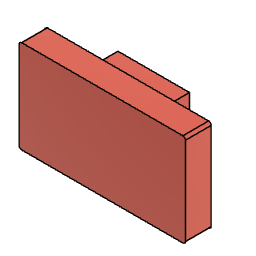
Switch Blocker v1 (Autodesk Fusion 360 design; units mm, degrees)
Autodesk Fusion 360 part; units mm, degrees
sketch "Sketch1" plane through (0, 0, 0) normal (0, 1, 0) x (1, 0, 0)
  line L0 (25.1, -18.075) -> (-6.2375, -18.075)
  line L1 (-6.7375, -17.575) -> (-6.7375, -0.525)
  line L2 (-6.2375, -0.025) -> (25.1, -0.025)
  line L3 (25.6, -17.575) -> (25.6, -0.525)
  line L4 (16.3813, -16) -> (16.3813, -2.1)
  line L5 (2.4813, -2.1) -> (16.3813, -2.1)
  line L6 (2.4813, -16) -> (2.4813, -2.1)
  line L7 (16.3813, -16) -> (2.4813, -16)
  arc A0 (-6.7375, -17.575) -> (-6.2375, -18.075) centre (-6.2375, -17.575) ccw
  arc A1 (-6.2375, -0.025) -> (-6.7375, -0.525) centre (-6.2375, -0.525) ccw
  arc A2 (25.1, -18.075) -> (25.6, -17.575) centre (25.1, -17.575) ccw
  arc A3 (25.6, -0.525) -> (25.1, -0.025) centre (25.1, -0.525) ccw
  line L8 (8.8409, -16) -> (8.8409, -18.075)
  line L9 (16.3813, -6.6239) -> (25.6, -6.6239)
  point P0 (25.6, -18.075)
  point P1 (-6.7375, -18.075)
  point P2 (25.6, -0.025)
  dimension "d39" = 0.5
  dimension "d40" = 0.5
  dimension "d41" = 0.5
  dimension "d42" = 0.5
  dimension "StemWidth" = 13.9
  dimension "StemHeight" = 13.9
  dimension "d62" = 2.075
  dimension "d63" = 9.2188
  constraint horizontal L0
  constraint vertical L1
  constraint horizontal L2
  constraint perpendicular L2 L3
  constraint coincident P1 L0
  constraint coincident P1 L1
  constraint tangent L0 A0
  constraint tangent L1 A0
  constraint tangent L1 A1
  constraint tangent L2 A1
  constraint coincident P0 L0
  constraint coincident P0 L3
  constraint tangent L0 A2
  constraint tangent L3 A2
  constraint coincident P2 L2
  constraint coincident P2 L3
  constraint tangent L2 A3
  constraint tangent L3 A3
  constraint parallel L3 L4
  constraint parallel L2 L5
  constraint parallel L1 L6
  constraint parallel L0 L7
  constraint coincident L7 L8.start
  constraint coincident L0 L8.end
  constraint perpendicular L0 L8
  constraint coincident L4 L9.start
  constraint coincident L3 L9.end
  constraint perpendicular L3 L9
  measures "d39" radius of A0
  measures "d40" radius of A1
  measures "d41" radius of A2
  measures "d42" radius of A3
  measures "StemWidth" distance of L4.start L4.end
  measures "StemHeight" distance of L4.start L6.start
  measures "d62" distance of L8.start L8.end
  measures "d63" distance of L9.start L9.end
extrude "Extrude1" add sketch "Sketch1" against normal blind 2
extrude "Extrude2" add sketch "Sketch1" along normal blind 5 contours L4 L5 L6 L7
extrude "Extrude3" add 1 faces at (4.2083, -2, 6.0417) along direction (0, -1, 0) blind 3
sketch "Sketch2" plane through (16.3813, 0, 0) normal (1, 0, 0) x (0, 1, 0)
  line L0 (0, 16) -> (0, 2.1)
  line L1 (0, 2.1) -> (5, 2.1)
  line L2 (5, 2.1) -> (5, 16)
  line L3 (5, 16) -> (0, 16)
  line L4 (0, 16) -> (0, 14)
  line L5 (0, 2.1) -> (0, 4.1)
  line L6 (0, 14) -> (1.5, 14)
  line L7 (0, 4.1) -> (1.5, 4.1)
  line L8 (1.5, 14) -> (3.5, 14)
  line L9 (3.5, 14) -> (3.5, 13)
  line L10 (3.5, 13) -> (1.5, 13)
  line L11 (1.5, 13) -> (1.5, 14)
  line L12 (1.5, 4.1) -> (3.5, 4.1)
  line L13 (3.5, 4.1) -> (3.5, 5.1)
  line L14 (3.5, 5.1) -> (1.5, 5.1)
  line L15 (1.5, 5.1) -> (1.5, 4.1)
  dimension "d16" = 2
  dimension "d17" = 2
  dimension "d18" = 1.5
  dimension "d19" = 1.5
  dimension "d20" = 2
  dimension "d21" = 1
  dimension "d22" = 2
  dimension "d23" = 1
  constraint coincident L0.start L3.end
  constraint perpendicular L3 L4
  constraint coincident L0.end L1.start
  constraint perpendicular L1 L5
  constraint perpendicular L4 L6
  constraint perpendicular L5 L7
  constraint horizontal L8
  constraint vertical L9
  constraint horizontal L10
  constraint vertical L11
  constraint horizontal L12
  constraint vertical L13
  constraint horizontal L14
  constraint vertical L15
  measures "d16" distance of L0.start L4.end
  measures "d17" distance of L0.end L5.end
  measures "d18" distance of L4.end L6.end
  measures "d19" distance of L5.end L7.end
  measures "d20" distance of L6.end L8.end
  measures "d21" distance of L6.end L10.end
  measures "d22" distance of L7.end L12.end
  measures "d23" distance of L7.end L14.end
extrude "Extrude4" add sketch "Sketch2" along normal blind 0.7 contours L8 L9 L10 L11 | L12 L13 L14 L15
draft "Draft1" angle -20 neutral plane through (16.3813, 1.5, 13) pull (0, -1, 0) 1 faces at (17.0813, 2.1667, 13.3333)
draft "Draft2" angle -20 neutral plane through (16.3813, 1.5, 5.1) pull (0, -1, 0) 1 faces at (17.0813, 2.1667, 4.4333)
sketch "Sketch3" plane through (2.4813, 0, 0) normal (-1, 0, 0) x (0, -1, 0)
  line L0 (0, 2.1) -> (0, 16)
  line L1 (0, 16) -> (-5, 16)
  line L2 (-5, 16) -> (-5, 2.1)
  line L3 (-5, 2.1) -> (0, 2.1)
  line L4 (-1.5, 13) -> (-1.5, 14)
  line L5 (-1.5, 14) -> (-3.5, 14)
  line L6 (-3.5, 14) -> (-3.5, 13)
  line L7 (-3.5, 13) -> (-1.5, 13)
  line L8 (-3.5, 5.1) -> (-1.5, 5.1)
  line L9 (-3.5, 4.1) -> (-3.5, 5.1)
  line L10 (-1.5, 4.1) -> (-3.5, 4.1)
  line L11 (-1.5, 5.1) -> (-1.5, 4.1)
extrude "Extrude5" add sketch "Sketch3" along normal blind 0.7 contours L4 L5 L6 L7 | L8 L9 L10 L11
draft "Draft3" angle -20 neutral plane through (2.4813, 1.5, 5.1) pull (0, -1, 0) 1 faces at (1.7813, 2.1667, 4.4333)
draft "Draft4" angle -20 neutral plane through (2.4813, 1.5, 13) pull (0, -1, 0) 1 faces at (1.7813, 2.1667, 13.3333)
sketch "Sketch4" plane through (0, 5, 0) normal (0, 1, 0) x (-1, 0, 0)
  line L0 (-16.3813, 16) -> (-16.3813, 2.1)
  line L1 (-16.3813, 2.1) -> (-2.4813, 2.1)
  line L2 (-2.4813, 2.1) -> (-2.4813, 16)
  line L3 (-2.4813, 16) -> (-16.3813, 16)
  line L4 (-14.3813, 4.1) -> (-4.4813, 4.1)
  line L5 (-4.4813, 4.1) -> (-4.4813, 14)
  line L6 (-4.4813, 14) -> (-14.3813, 14)
  line L7 (-14.3813, 14) -> (-14.3813, 4.1)
extrude "Extrude6" cut sketch "Sketch4" against normal blind 6 contours L4 L5 L6 L7
equation "CapWidth = ( Spacing * Width ) - Gap"
equation "CapHeight = ( Spacing * Height ) - Gap"
equation "d12 = PlateToPCB"
equation "d14 = BlockerHeight"
equation "d16 = DistanceToTooth"
equation "d17 = DistanceToTooth"
equation "d18 = PlateThickness"
equation "d19 = PlateThickness"
equation "d24 = ToothThickness"
equation "d26 = -ToothDraftAngle"
equation "d28 = -ToothDraftAngle"
equation "d30 = ToothThickness"
equation "d32 = -ToothDraftAngle"
equation "d34 = -ToothDraftAngle"
equation "d36 = -WallThickness"
equation "d37 = -( ( PlateToPCB + BlockerHeight ) - WallThickness )"
equation "d39 = BlockerRadius"
equation "d40 = BlockerRadius"
equation "d41 = BlockerRadius"
equation "d42 = BlockerRadius"
equation "Width = 1.75" comment "In Switch Units \"U\""
equation "Spacing = 19.05 mm"
equation "Height = 1" comment "In Switch Units \"U\""
equation "SwitchCutH = 14 mm" comment "Switch Cutout Height"
equation "SwitchCutW = 14 mm" comment "Switch Cutout Width"
equation "PlateThickness = 1.5 mm"
equation "PlateToPCB = 5 mm"
equation "BlockerHeight = 3 mm"
equation "BlockerRadius = 0.5 mm"
equation "Gap = 1 mm" comment "Total Gap"
equation "WallThickness = 2 mm"
equation "DistanceToTooth = 2 mm"
equation "ToothLength = 2 mm"
equation "ToothWidth = 1 mm"
equation "ToothThickness = 0.7 mm"
equation "ToothDraftAngle = 20"
equation "StemWidth = SwitchCutW - 0.1 mm"
equation "StemHeight = SwitchCutH - 0.1 mm"
equation "d62 = ( ( ( Spacing * Height ) - Gap ) - ( SwitchCutH - 0.1 mm ) ) / 2"
equation "d63 = ( ( ( Spacing * Width ) - Gap ) - ( SwitchCutW - 0.1 mm ) ) / 2"
named bodies: "Switch Blocker"
